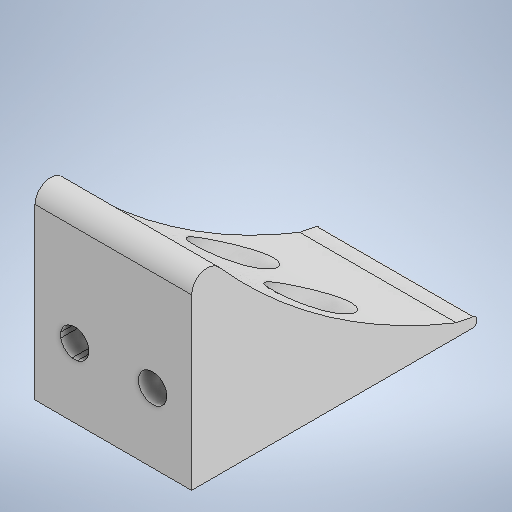
# Autodesk Inventor part: intake ramp piece
Saved by Autodesk Inventor 2025.1 (Build 291241020, 241B)
## iProperties
Created: 2024-12-04
Part Number: intake ramp piece
Material: Generic
Document SubType Name: Modeling
Designer: Hunter Mathis
Density: 1 g/cm^3
Appearance: Default
Author: Hunter Mathis
## iProperties of the stored document Round intake ramp piece_3DPrint.ipt
Created: 2024-12-08
Part Number: Round intake ramp piece_3DPrint
Material: Generic
Document SubType Name: Modeling
Designer: AtuStem
Density: 1 g/cm^3
Appearance: Default
Author: AtuStem
Autodesk Inventor part; units mm, degrees
ref_plane "YZ Plane" through (0, 0, 0) normal (1, 0, 0) x (0, 1, 0)
ref_plane "XZ Plane" through (0, 0, 0) normal (0, 1, 0) x (-1, 0, 0)
ref_plane "XY Plane" through (0, 0, 0) normal (0, 0, 1) x (1, 0, 0)
sketch "Sketch24" plane through (0, 0, 0) normal (0, 0, 1) x (1, 0, 0)
  line L0 (0, 0) -> (177.8, 0)
  line L1 (177.8, 0) -> (177.8, 33.0962)
  line L2 (177.8, 33.0962) -> (0, 33.0962)
  line L3 (0, 33.0962) -> (0, 0)
  line L4 (88.9, 33.0962) -> (88.9, 0)
  line L5 (88.9, 0) -> (88.9, 7.3914)
  line L6 (88.9, 7.3914) -> (95.25, 7.3914)
  line L7 (94.488, 11.9634) -> (96.012, 11.9634)
  line L8 (97.536, 10.4394) -> (97.536, 8.9154)
  line L9 (96.012, 7.3914) -> (94.488, 7.3914)
  line L10 (92.964, 8.9154) -> (92.964, 10.4394)
  arc A0 (94.488, 11.9634) -> (92.964, 10.4394) centre (94.488, 10.4394) ccw
  arc A1 (97.536, 10.4394) -> (96.012, 11.9634) centre (96.012, 10.4394) ccw
  arc A2 (96.012, 7.3914) -> (97.536, 8.9154) centre (96.012, 8.9154) ccw
  arc A3 (92.964, 8.9154) -> (94.488, 7.3914) centre (94.488, 8.9154) ccw
  arc A4 (110.236, 10.4394) -> (108.712, 11.9634) centre (108.712, 10.4394) ccw
  arc A5 (108.712, 7.3914) -> (110.236, 8.9154) centre (108.712, 8.9154) ccw
  line L11 (108.712, 7.3914) -> (107.188, 7.3914)
  line L12 (105.664, 8.9154) -> (105.664, 10.4394)
  arc A6 (107.188, 11.9634) -> (105.664, 10.4394) centre (107.188, 10.4394) ccw
  arc A7 (105.664, 8.9154) -> (107.188, 7.3914) centre (107.188, 8.9154) ccw
  line L13 (107.188, 11.9634) -> (108.712, 11.9634)
  line L14 (110.236, 10.4394) -> (110.236, 8.9154)
  arc A8 (84.836, 10.4394) -> (83.312, 11.9634) centre (83.312, 10.4394) ccw
  arc A9 (83.312, 7.3914) -> (84.836, 8.9154) centre (83.312, 8.9154) ccw
  line L15 (83.312, 7.3914) -> (81.788, 7.3914)
  line L16 (80.264, 8.9154) -> (80.264, 10.4394)
  arc A10 (81.788, 11.9634) -> (80.264, 10.4394) centre (81.788, 10.4394) ccw
  arc A11 (80.264, 8.9154) -> (81.788, 7.3914) centre (81.788, 8.9154) ccw
  line L17 (81.788, 11.9634) -> (83.312, 11.9634)
  line L18 (84.836, 10.4394) -> (84.836, 8.9154)
  arc A12 (122.936, 10.4394) -> (121.412, 11.9634) centre (121.412, 10.4394) ccw
  arc A13 (121.412, 7.3914) -> (122.936, 8.9154) centre (121.412, 8.9154) ccw
  line L19 (121.412, 7.3914) -> (119.888, 7.3914)
  line L20 (118.364, 8.9154) -> (118.364, 10.4394)
  arc A14 (119.888, 11.9634) -> (118.364, 10.4394) centre (119.888, 10.4394) ccw
  arc A15 (118.364, 8.9154) -> (119.888, 7.3914) centre (119.888, 8.9154) ccw
  line L21 (119.888, 11.9634) -> (121.412, 11.9634)
  line L22 (122.936, 10.4394) -> (122.936, 8.9154)
  arc A16 (72.136, 10.4394) -> (70.612, 11.9634) centre (70.612, 10.4394) ccw
  arc A17 (70.612, 7.3914) -> (72.136, 8.9154) centre (70.612, 8.9154) ccw
  line L23 (70.612, 7.3914) -> (69.088, 7.3914)
  line L24 (67.564, 8.9154) -> (67.564, 10.4394)
  arc A18 (69.088, 11.9634) -> (67.564, 10.4394) centre (69.088, 10.4394) ccw
  arc A19 (67.564, 8.9154) -> (69.088, 7.3914) centre (69.088, 8.9154) ccw
  line L25 (69.088, 11.9634) -> (70.612, 11.9634)
  line L26 (72.136, 10.4394) -> (72.136, 8.9154)
  arc A20 (135.636, 10.4394) -> (134.112, 11.9634) centre (134.112, 10.4394) ccw
  arc A21 (134.112, 7.3914) -> (135.636, 8.9154) centre (134.112, 8.9154) ccw
  line L27 (134.112, 7.3914) -> (132.588, 7.3914)
  line L28 (131.064, 8.9154) -> (131.064, 10.4394)
  arc A22 (132.588, 11.9634) -> (131.064, 10.4394) centre (132.588, 10.4394) ccw
  arc A23 (131.064, 8.9154) -> (132.588, 7.3914) centre (132.588, 8.9154) ccw
  line L29 (132.588, 11.9634) -> (134.112, 11.9634)
  line L30 (135.636, 10.4394) -> (135.636, 8.9154)
  arc A24 (59.436, 10.4394) -> (57.912, 11.9634) centre (57.912, 10.4394) ccw
  arc A25 (57.912, 7.3914) -> (59.436, 8.9154) centre (57.912, 8.9154) ccw
  line L31 (57.912, 7.3914) -> (56.388, 7.3914)
  line L32 (54.864, 8.9154) -> (54.864, 10.4394)
  arc A26 (56.388, 11.9634) -> (54.864, 10.4394) centre (56.388, 10.4394) ccw
  arc A27 (54.864, 8.9154) -> (56.388, 7.3914) centre (56.388, 8.9154) ccw
  line L33 (56.388, 11.9634) -> (57.912, 11.9634)
  line L34 (59.436, 10.4394) -> (59.436, 8.9154)
  arc A28 (148.336, 10.4394) -> (146.812, 11.9634) centre (146.812, 10.4394) ccw
  arc A29 (146.812, 7.3914) -> (148.336, 8.9154) centre (146.812, 8.9154) ccw
  line L35 (146.812, 7.3914) -> (145.288, 7.3914)
  line L36 (143.764, 8.9154) -> (143.764, 10.4394)
  arc A30 (145.288, 11.9634) -> (143.764, 10.4394) centre (145.288, 10.4394) ccw
  arc A31 (143.764, 8.9154) -> (145.288, 7.3914) centre (145.288, 8.9154) ccw
  line L37 (145.288, 11.9634) -> (146.812, 11.9634)
  line L38 (148.336, 10.4394) -> (148.336, 8.9154)
  arc A32 (46.736, 10.4394) -> (45.212, 11.9634) centre (45.212, 10.4394) ccw
  arc A33 (45.212, 7.3914) -> (46.736, 8.9154) centre (45.212, 8.9154) ccw
  line L39 (45.212, 7.3914) -> (43.688, 7.3914)
  line L40 (42.164, 8.9154) -> (42.164, 10.4394)
  arc A34 (43.688, 11.9634) -> (42.164, 10.4394) centre (43.688, 10.4394) ccw
  arc A35 (42.164, 8.9154) -> (43.688, 7.3914) centre (43.688, 8.9154) ccw
  line L41 (43.688, 11.9634) -> (45.212, 11.9634)
  line L42 (46.736, 10.4394) -> (46.736, 8.9154)
  arc A36 (161.036, 10.4394) -> (159.512, 11.9634) centre (159.512, 10.4394) ccw
  arc A37 (159.512, 7.3914) -> (161.036, 8.9154) centre (159.512, 8.9154) ccw
  line L43 (159.512, 7.3914) -> (157.988, 7.3914)
  line L44 (156.464, 8.9154) -> (156.464, 10.4394)
  arc A38 (157.988, 11.9634) -> (156.464, 10.4394) centre (157.988, 10.4394) ccw
  arc A39 (156.464, 8.9154) -> (157.988, 7.3914) centre (157.988, 8.9154) ccw
  line L45 (157.988, 11.9634) -> (159.512, 11.9634)
  line L46 (161.036, 10.4394) -> (161.036, 8.9154)
  circle A40 centre (120.65, 9.6774) radius 2.3241
  point P0 (95.25, 9.6774)
  point P1 (95.25, 7.3914)
  point P2 (107.95, 7.3914)
  point P3 (107.95, 9.6774)
  point P4 (107.95, 7.3914)
  point P5 (82.55, 7.3914)
  point P6 (82.55, 9.6774)
  point P7 (82.55, 7.3914)
  point P8 (120.65, 7.3914)
  point P9 (120.65, 7.3914)
  point P10 (69.85, 7.3914)
  point P11 (69.85, 9.6774)
  point P12 (69.85, 7.3914)
  point P13 (133.35, 7.3914)
  point P14 (133.35, 9.6774)
  point P15 (133.35, 7.3914)
  point P16 (57.15, 7.3914)
  point P17 (57.15, 9.6774)
  point P18 (57.15, 7.3914)
  point P19 (146.05, 7.3914)
  point P20 (146.05, 9.6774)
  point P21 (146.05, 7.3914)
  point P22 (44.45, 7.3914)
  point P23 (44.45, 9.6774)
  point P24 (44.45, 7.3914)
  point P25 (158.75, 7.3914)
  point P26 (158.75, 9.6774)
  point P27 (158.75, 7.3914)
  point P28 (122.936, 10.0965)
  point P29 (121.0691, 11.9634)
  point P30 (120.2309, 11.9634)
  point P31 (118.364, 10.0965)
  point P32 (118.364, 9.2583)
  point P33 (120.2309, 7.3914)
  point P34 (121.0691, 7.3914)
  point P35 (122.936, 9.2583)
  dimension "d106" = 177.8
  dimension "d107" = 33.0962
  dimension "d119" = 7.3914
  dimension "d120" = 6.35
  dimension "d121" = 1.524
  dimension "d180" = 12.7
  dimension "d244" = 4.6482
  constraints: 94 end point, 80 point on circle, 41 centre point, 8 tangent, 4 parallel, 3 equal radius, 3 horizontal, 3 midpoint, 3 perpendicular, 1 coincident, 1 point on line, 207 other
  measures "d106" distance of L2.end L1.end
  measures "d107" distance of L0.end L1.end
  measures "d119" distance of L4.end L5.end
  measures "d120" distance of L5.end L6.end
  measures "d121" radius of A0
  measures "d180" distance of A1.centre A4.centre
  measures "d244" diameter of A40
sketch "Sketch26" plane through (0, 0, 0) normal (1, 0, 0) x (0, 1, 0)
  line L0 (0, 0) -> (0, -44.45)
  line L1 (33.0962, 0) -> (0, 0) projected
  arc A0 (33.0962, 0) -> (0, -44.45) centre (95.48, -80.9954) ccw
  dimension "d108" = 44.45
  dimension "d109" = 102.235
  constraints: 2 end point, 2 point on circle, 1 centre point, 1 vertical
  measures "d108" distance of L0.start L0.end
  measures "d109" radius of A0
extrude "Extrusion23" add sketch "Sketch26" along normal blind 177.8
sketch "Sketch27" plane through (0, 0, 0) normal (0, 0, 1) x (1, 0, 0)
  line L0 (0, 0) -> (44.45, 0)
  line L1 (0, 0) -> (177.8, 0) projected
  line L2 (44.45, 0) -> (44.45, 33.0962)
  line L3 (0, 33.0962) -> (177.8, 33.0962) projected
  arc A0 (0, 0) -> (44.45, 33.0962) centre (-36.5454, 95.48) ccw
  line L4 (0, 33.0962) -> (0, 0) projected
  line L5 (0, 0) -> (0, 33.0962)
  line L6 (0, 33.0962) -> (44.45, 33.0962)
  line L7 (0, 33.0962) -> (-19.05, 33.0962)
  line L8 (-19.05, 33.0962) -> (-19.05, 0)
  line L9 (-19.05, 0) -> (0, 0)
  line L10 (0, 0) -> (0, 33.0962)
  dimension "d112" = 44.45
  dimension "d113" = 102.235
  dimension "d114" = 19.05
  constraints: 16 end point, 3 equal length, 3 perpendicular, 2 point on circle, 2 point on line, 1 centre point, 1 horizontal
  measures "d112" distance of L0.start L0.end
  measures "d113" radius of A0
  measures "d114" distance of L9.end L8.end
revolve "Revolution1" [suppressed]
ref_plane "Work Plane3" through (88.9, 33.0962, 0) normal (-1, 0, 0) x (0, -1, 0)
mirror "Mirror1" [suppressed]
ref_plane "Work Plane4" through (44.45, 32.1705, -50.8) normal (0, 0, 1) x (1, 0, 0)
sketch "Sketch28" plane through (44.45, 32.1705, -50.8) normal (0, 0, 1) x (1, 0, 0)
  line L0 (27.686, -23.2551) -> (27.686, -21.7311) projected
  arc A0 (27.686, -21.7311) -> (26.162, -20.2071) centre (26.162, -21.7311) ccw projected
  line L1 (26.162, -20.2071) -> (24.638, -20.2071) projected
  arc A1 (24.638, -20.2071) -> (23.114, -21.7311) centre (24.638, -21.7311) ccw projected
  line L2 (23.114, -21.7311) -> (23.114, -23.2551) projected
  arc A2 (23.114, -23.2551) -> (24.638, -24.7791) centre (24.638, -23.2551) ccw projected
  line L3 (24.638, -24.7791) -> (26.162, -24.7791) projected
  arc A3 (26.162, -24.7791) -> (27.686, -23.2551) centre (26.162, -23.2551) ccw projected
  line L4 (65.786, -23.2551) -> (65.786, -21.7311) projected
  arc A4 (65.786, -21.7311) -> (64.262, -20.2071) centre (64.262, -21.7311) ccw projected
  line L5 (64.262, -20.2071) -> (62.738, -20.2071) projected
  arc A5 (62.738, -20.2071) -> (61.214, -21.7311) centre (62.738, -21.7311) ccw projected
  line L6 (61.214, -21.7311) -> (61.214, -23.2551) projected
  arc A6 (61.214, -23.2551) -> (62.738, -24.7791) centre (62.738, -23.2551) ccw projected
  line L7 (62.738, -24.7791) -> (64.262, -24.7791) projected
  arc A7 (64.262, -24.7791) -> (65.786, -23.2551) centre (64.262, -23.2551) ccw projected
  line L8 (91.186, -23.2551) -> (91.186, -21.7311) projected
  arc A8 (91.186, -21.7311) -> (89.662, -20.2071) centre (89.662, -21.7311) ccw projected
  line L9 (89.662, -20.2071) -> (88.138, -20.2071) projected
  arc A9 (88.138, -20.2071) -> (86.614, -21.7311) centre (88.138, -21.7311) ccw projected
  line L10 (86.614, -21.7311) -> (86.614, -23.2551) projected
  arc A10 (86.614, -23.2551) -> (88.138, -24.7791) centre (88.138, -23.2551) ccw projected
  line L11 (88.138, -24.7791) -> (89.662, -24.7791) projected
  arc A11 (89.662, -24.7791) -> (91.186, -23.2551) centre (89.662, -23.2551) ccw projected
  line L12 (2.286, -23.2551) -> (2.286, -21.7311) projected
  arc A12 (2.286, -21.7311) -> (0.762, -20.2071) centre (0.762, -21.7311) ccw projected
  line L13 (0.762, -20.2071) -> (-0.762, -20.2071) projected
  arc A13 (-0.762, -20.2071) -> (-2.286, -21.7311) centre (-0.762, -21.7311) ccw projected
  line L14 (-2.286, -21.7311) -> (-2.286, -23.2551) projected
  arc A14 (-2.286, -23.2551) -> (-0.762, -24.7791) centre (-0.762, -23.2551) ccw projected
  line L15 (-0.762, -24.7791) -> (0.762, -24.7791) projected
  arc A15 (0.762, -24.7791) -> (2.286, -23.2551) centre (0.762, -23.2551) ccw projected
  line L16 (0, -32.1705) -> (0, 0.196) projected
  line L17 (88.9, -22.4931) -> (76.2, -22.4931)
  circle A16 centre (76.2, -22.4931) radius 4.1275
  point P0 (-44.45, -32.1705)
  dimension "d247" = 12.7
  dimension "d248" = 8.255
  constraints: 2 end point, 1 centre point, 1 coincident, 1 horizontal
  measures "d247" distance of L17.start L17.end
  measures "d248" diameter of A16
sketch3d "3D Sketch1"
hole "Hole1" at (133.35, 9.6774, -25.4084) direction (0, 0, 1) diameter 4.6482 end through all start extended yes counterbore diameter 8.255 counterbore depth 5.8928
hole "Hole2" at (107.95, 9.6774, -25.4084) direction (0, 0, 1) diameter 4.6482 end through all start extended yes counterbore diameter 8.255 counterbore depth 5.8928
hole "Hole3" at (69.85, 9.6774, -25.4084) direction (0, 0, 1) diameter 4.6482 end through all start extended yes counterbore diameter 8.255 counterbore depth 5.8928
hole "Hole4" at (44.45, 9.6774, -25.4084) direction (0, 0, 1) diameter 4.6482 end through all start extended yes counterbore diameter 8.255 counterbore depth 5.8928
ref_plane "Work Plane5" through (2.0079, 0, -0.381) normal (0, -1, 0) x (1, 0, 0)
sketch "Sketch32" plane through (44.45, 0, -44.45) normal (0, -1, 0) x (1, 0, 0)
  arc A0 (-44.4489, 44.1317) -> (0, 0) centre (0, 44.45) ccw projected
  arc A1 (-44.45, 44.45) -> (0, 0) centre (0, 44.45) ccw
  arc A2 (88.9, 0) -> (133.3489, 44.1317) centre (88.9, 44.45) ccw projected
  arc A3 (88.9, 0) -> (133.3489, 44.1317) centre (88.9, 44.45) ccw
  line L0 (0, 0) -> (88.9, 0) projected
  line L1 (88.9, 0) -> (0, 0)
  arc A4 (88.9, 0) -> (133.3489, 44.1317) centre (88.9, 44.45) ccw
  arc A5 (88.9, 0) -> (133.3489, 44.1317) centre (88.9, 44.45) ccw
  line L2 (0, 0) -> (0, 12.0815) projected
  arc A6 (-44.4489, 44.1317) -> (0, 0) centre (0, 44.45) ccw
  line L3 (-43.5698, 44.45) -> (132.4698, 44.45) projected
  line L4 (132.4698, 44.45) -> (-43.5698, 44.45)
  line L5 (0, 0) -> (88.9, 0)
  arc A7 (-43.5698, 44.45) -> (-44.4489, 44.1317) centre (-43.5012, 42.8875) ccw
  arc A8 (133.3489, 44.1317) -> (132.4698, 44.45) centre (132.2102, 42.3602) ccw
  constraints: 15 point on circle, 7 centre point, 6 end point, 3 collinear
extrude "Extrusion26" [suppressed]
fillet "Fillet21" radius 0.254 1 edges at (88.9, 0, -44.45)
ref_plane "Work Plane11" through (44.45, 32.1705, 0) normal (0, 0, 1) x (1, 0, 0)
sketch "Sketch33" plane through (44.45, 32.1705, 0) normal (0, 0, 1) x (1, 0, 0)
  line L0 (-44.45, 0) -> (133.35, 0) projected
  line L1 (0, 0) -> (19.05, 0)
  line L2 (19.05, 0) -> (19.05, -33.5816)
  line L3 (0, -33.5816) -> (88.9, -33.5816) projected
  line L4 (69.7162, -33.5816) -> (69.7162, 0)
  line L5 (69.7162, 0) -> (19.05, 0)
  line L6 (19.05, 0) -> (19.05, 3.1547)
  line L7 (19.05, 3.1547) -> (69.7162, 3.1547)
  line L8 (69.7162, 3.1547) -> (69.7162, 0)
  line L9 (19.05, 0) -> (69.7162, 0)
  point P0 (-44.45, -32.1705)
  point P1 (88.9, 0)
  point P2 (69.7162, 0)
  point P3 (69.7162, 0)
  dimension "d185" = 19.05
  constraints: 16 end point, 4 perpendicular, 4 point on line, 2 equal length, 1 vertical
  measures "d185" distance of L1.start L1.end
extrude "Extrusion27" cut sketch "Sketch33" along normal through all both and the other way through all
sketch "Sketch36" plane through (44.45, -1.4111, -44.45) normal (0, -1, 0) x (1, 0, 0)
  point P0 (-44.45, 44.45)
sketch "Sketch37" plane through (177.8, 0, -43.1007) normal (0, -1, 0) x (1, 0, 0)
  line L0 (-29.7024, 55.8355) -> (18.8644, 55.8355)
  line L1 (18.8644, 55.8355) -> (18.8644, -23.5807)
  line L2 (18.8644, -23.5807) -> (-29.7024, -23.5807)
  line L3 (-29.7024, 55.8355) -> (-38.095, 55.8355)
  line L4 (-38.095, 55.8355) -> (-38.095, -23.5807)
  line L5 (-38.095, -23.5807) -> (-29.7024, -23.5807)
  point P0 (-177.8, 43.1007)
  constraints: 12 end point, 2 horizontal, 2 perpendicular, 1 collinear, 1 parallel
extrude "Extrusion28" cut sketch "Sketch37" against normal through all
ref_plane "Work Plane6" through (88.9, 0, 0) normal (1, 0, 0) x (0, 0, -1)
mirror "Mirror2" about plane through (88.9, 0, 0) normal (1, 0, 0) of "Extrusion28"
ref_plane "Work Plane12" through (114.1662, 0, 0) normal (0, 0, 1) x (1, 0, 0)
ref_plane "Work Plane13" through (114.1662, 17.603, 24.13) normal (0, -1, 0) x (1, 0, 0)
fillet "Fillet25" radius 2.54 2 edges at (126.9356, 33.0962, 0) (50.7975, 33.0962, 0)
sketch "Sketch40" plane through (63.5, 0, 0) normal (0, 0, 1) x (1, 0, 0)
  line L0 (8.2246, 40.0148) -> (-39.0885, 40.0148)
  line L1 (-39.0885, 40.0148) -> (-39.0885, -10.9894)
  line L2 (-39.0885, -10.9894) -> (8.2246, -10.9894)
  line L3 (8.2246, -10.9894) -> (8.2246, 40.0148)
  point P0 (-63.5, 0)
  constraints: 8 end point, 2 parallel, 1 horizontal, 1 perpendicular
extrude "Extrusion31" cut sketch "Sketch40" along normal through all both and the other way through all
sketch "Sketch41" plane through (114.1662, 0, -43.1007) normal (0, -1, 0) x (1, 0, 0)
  line L0 (25.5388, 0) -> (25.5388, 43.1007) projected
  line L1 (0, 43.1007) -> (25.5388, 43.1007) projected
  line L2 (0, 43.1007) -> (0, 0) projected
  line L3 (25.5388, 0) -> (0, 0) projected
  point P0 (-114.1662, 43.1007)
sketch "Sketch42" plane through (139.705, 0, 0) normal (1, 0, 0) x (0, 0, -1)
  line L0 (0, 0) -> (0, 26.0354) projected
  line L1 (43.1007, 0) -> (0, 0) projected
  arc A0 (43.1007, 0) -> (43.1947, 0.49) centre (43.1007, 0.254) ccw projected
  arc A1 (4.4419, 27.7189) -> (43.1947, 0.49) centre (80.9954, 95.48) ccw projected
  arc A2 (4.4419, 27.7189) -> (0, 26.0354) centre (2.54, 26.0354) ccw projected
  line L2 (0, 0) -> (0, -1.5875)
  line L3 (0, -1.5875) -> (54.2562, -1.5875)
  line L4 (54.2562, -1.5875) -> (43.1477, 0.5036)
  point P0 (43.1719, 0.4991)
  dimension "d229" = 1.5875
  constraints: 6 end point, 1 perpendicular, 1 point on circle, 1 tangent, 1 vertical
  measures "d229" distance of L0.start L2.end
extrude "Extrusion32" add sketch "Sketch42" against normal up to surface (25.5388 mm away) contours L1 A0 A1 L4 L3 L2
fillet "Fillet28" radius 0.7937 1 edges at (126.9356, -1.5875, -54.2562)
extrude "Extrusion36" cut sketch "Sketch24" against normal blind 33.3375 contours L22 A40 L19 L20 L21
hole "Hole5" at (120.65, 9.6774, -50.8) direction (0, 0, 1) diameter 8.255 depth 32.3342 tip angle 118 start extended yes
body "Solid2"
